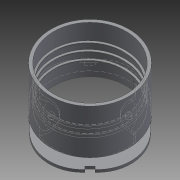
# Autodesk Inventor part: DiffuserCoupler
Saved by Autodesk Inventor 2014 SP2 (Build 180246200, 246)
## iProperties
Created: 2014-02-09
Part Number: DiffuserCoupler
Material: Generic
Document SubType Name: Modeling
Designer: jkao
Density: 1 g/cm^3
Appearance: Default
Author: jkao
Autodesk Inventor part; units mm, degrees
ref_plane "YZ Plane" through (0, 0, 0) normal (1, 0, 0) x (0, 1, 0)
ref_plane "XZ Plane" through (0, 0, 0) normal (0, 1, 0) x (-1, 0, 0)
ref_plane "XY Plane" through (0, 0, 0) normal (0, 0, 1) x (1, 0, 0)
sketch "Collar Profile" plane through (0, 0, 0) normal (0, 0, 1) x (1, 0, 0)
  circle A0 centre (0, 0) radius 13.75
  circle A1 centre (0, 0) radius 14.75
  dimension "collarInnerDiameter" = 27.5
  dimension "d74" = 29.5
  constraints: 2 centre point
  measures "collarInnerDiameter" diameter of A0
  measures "d74" diameter of A1
extrude "Collar" add sketch "Collar Profile" along normal blind 18.5
sketch "Thread Profile" plane through (0, 0, 0) normal (0, 1, 0) x (-1, 0, 0)
  line L0 (0, 27.549911) -> (0, -8)
  line L1 (13.75, 13) -> (13.15, 12.915052)
  line L2 (13.75, 13) -> (13.75, 12)
  line L3 (13.15, 12.915052) -> (13.15, 12.715052)
  line L4 (13.75, 12) -> (13.15, 12.715052)
  line L5 (13.75, 12) -> (14.386651, 12) construction
  line L6 (-14.75, 0) -> (14.75, 0)
  point P0 (0, 0)
  dimension "d98" = 1
  dimension "d99" = 130
  dimension "d100" = 12
  dimension "d125" = 0.2
  dimension "d127" = 0.6
  dimension "d128" = 13.75
  constraints: 12 end point, 2 vertical, 1 horizontal
  measures "d98" distance of L1.start L2.end
  measures "d99" angle of L5 L4
  measures "d100" distance between parallel lines of L5 L6
  measures "d125" distance of L1.end L3.end
  measures "d127" distance between parallel lines of L3 L2
  measures "d128" distance between parallel lines of L0 L2
coil "Diffuser Thread" sketch "Thread Profile" operation add axis through (0, 0, 27.549911) along (0, 0, -1) pitch 3 turns 2.5 hand right
fillet "Fillet3" radius 3 1 edges at (-13.15, 0, 12.8151)
sketch "Screw Tab Profile" plane through (0, 0, 0) normal (0, 0, -1) x (-1, 0, 0)
  arc A0 (-13.75, 0) -> (-12.213593, -6.315905) centre (0, 0) ccw
  arc A1 (-13.249986, 6.48077) -> (13.249999, -6.480742) centre (0, 0) ccw
  arc A2 (-13.249986, -6.48077) -> (-12.213593, 6.315905) centre (-13.749609, 0) ccw
  arc A3 (13.249999, 6.480742) -> (12.213635, 6.315824) centre (13.749984, 0) ccw
  line L0 (-14.5, 18.75) -> (-1.25, 18.75)
  line L1 (14.5, -18.75) -> (1.25, -18.75)
  arc A4 (-12.213593, 6.315905) -> (-13.249986, 6.48077) centre (-13.749609, 0) ccw
  arc A5 (12.213635, 6.315824) -> (12.213635, -6.315824) centre (13.749984, 0) ccw
  arc A6 (-12.213593, 6.315905) -> (-13.75, 0) centre (0, 0) ccw
  arc A7 (-12.213593, -6.315905) -> (12.213635, -6.315824) centre (0, 0) ccw
  arc A8 (12.213635, 6.315824) -> (-12.213593, 6.315905) centre (0, 0) ccw
  arc A9 (12.213635, -6.315824) -> (12.213635, 6.315824) centre (0, 0) ccw
  arc A10 (12.213635, -6.315824) -> (13.249999, -6.480742) centre (13.749984, 0) ccw
  arc A11 (13.249999, 6.480742) -> (-13.249986, 6.48077) centre (0, 0) ccw
  arc A12 (13.249999, -6.480742) -> (13.249999, 6.480742) centre (0, 0) ccw
  line L2 (-1.25, 18.75) -> (-1.25, 17.65)
  line L3 (1.25, 18.75) -> (1.25, 17.65)
  line L4 (1.25, 17.65) -> (-1.25, 17.65)
  line L5 (1.25, 18.75) -> (14.5, 18.75)
  line L6 (-1.25, 18.75) -> (1.25, 18.75)
  line L7 (-1.25, -18.75) -> (-1.25, -17.65)
  line L8 (1.25, -18.75) -> (1.25, -17.65)
  line L9 (1.25, -17.65) -> (-1.25, -17.65)
  line L10 (1.25, -18.75) -> (-1.25, -18.75)
  line L11 (-1.25, -18.75) -> (-14.5, -18.75)
  line L12 (14.5, 18.75) -> (14.5, -18.75)
  line L13 (-14.5, 18.75) -> (-14.5, -18.75)
  point P0 (-9.249609, 0)
  point P1 (9.249984, 0)
  point P2 (-0.0003, 16.4)
  point P3 (0, -16.4)
  dimension "d103" = 6.5
  dimension "d105" = 6.5
  dimension "d108" = 4.5
  dimension "d109" = 4.5
  dimension "d129" = 29.5
  dimension "d145" = 18.75
  dimension "d148" = 18.75
  dimension "d149" = 1.1
  dimension "d152" = 2.5
  dimension "d153" = 29
  dimension "d156" = 14.5
  dimension "d157" = 14.5
  constraints: 30 point on circle, 28 end point, 13 centre point, 11 parallel, 3 horizontal, 2 perpendicular
  measures "d103" radius of A2
  measures "d105" radius of A3
  measures "d108" distance of A2.centre point (-9.25, 0)
  measures "d109" distance of A3.centre point (9.25, 0)
  measures "d129" diameter of A1
  measures "d145" distance from line of L0 point (0, 0)
  measures "d148" distance from line of L1 point (0, 0)
  measures "d149" distance of L0.end L2.end
  measures "d152" distance between parallel lines of L3 L2
  measures "d153" distance between parallel lines of L12 L13
  measures "d156" distance from line of L13 A0.centre
  measures "d157" distance from line of L12 A0.centre
extrude "Tabs" add sketch "Screw Tab Profile" against normal blind 1 contours A6 A2 A0 | A0 A2 A1 L13 A4 A6 | A7 A10 A1 A2 | A4 A11 A3 A8 | A1 A12 L12 L1 L8 L9 L7 L11 L13 | A5 A9 | A9 A3 A12 L12 A10 | A1 L13 L0 L2 L4 L3 L5 L12 A12 A11 | A1 L13 | L12 A12
hole "Screw Holes" at (9.249609, 0, 0) at (-9.249984, 0, 0) direction (0, 0, 1) diameter 1.7 end through all clearance for "Socket Head Cap Screw" size "M1.6" standard "Ansi Metric M Profile"
fillet "Fillet6" radius 2.5 5 edges at (13.3604, 3.25, 1) (13.3604, -3.25, 1) (-13.75, 0, 1) (12.2136, -6.3159, 0.5) (12.2136, 6.3159, 0.5)
fillet "Fillet7" radius 12.75 4 edges at (-14.5, -18.75, 0.5) (14.5, -18.75, 0.5) (14.5, 18.75, 0.5) (-14.5, 18.75, 0.5)
equation "\"d128\" = 0.5 * collarInnerDiameter"
body "Solid3"
